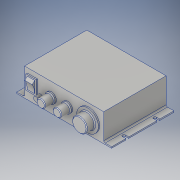
# Autodesk Inventor part: AmpLP2020A
Saved by Autodesk Inventor 2017 (Build 210142000, 142)
## iProperties
Created: 2018-08-06
Part Number: AmpLP2020A
Material: Aluminum 6061
Document SubType Name: Modeling
Designer: Jake
Density: 2.7 g/cm^3
Appearance: Aluminum - Flat
Author: Jake
Autodesk Inventor part; units mm, degrees
ref_plane "YZ Plane" through (0, 0, 0) normal (1, 0, 0) x (0, 1, 0)
sketch "Sketch1" plane through (0, 0, 0) normal (0, 1, 0) x (-1, 0, 0)
  line L0 (70, -46) -> (-70, -46)
  line L1 (-70, -46) -> (-70, 46)
  line L2 (-70, 46) -> (70, 46)
  line L3 (70, 46) -> (70, -46)
  point P0 (0, 0)
  point P1 (0, -46)
  point P2 (-70, 0)
  dimension "d0" = 92
  dimension "d1" = 140
  constraints: 8 end point, 2 midpoint, 2 parallel, 1 horizontal, 1 horizontal alignment, 1 perpendicular, 1 vertical alignment
  measures "d0" distance of L0.end L1.end
  measures "d1" distance of L0.start L0.end
extrude "Extrusion1" add sketch "Sketch1" along normal blind 2
sketch "Sketch2" plane through (0, 2, 0) normal (0, 1, 0) x (1, 0, 0)
  line L0 (70, 46) -> (-70, 46) projected
  line L1 (-70, 46) -> (-70, -46) projected
  line L2 (-70, -46) -> (70, -46) projected
  line L3 (70, -46) -> (70, 46) projected
  line L4 (70, 46) -> (-70, 46) projected
  line L5 (-70, -46) -> (70, -46) projected
  line L6 (-58.5, 46) -> (58.5, 46)
  line L7 (58.5, 46) -> (58.5, -46)
  line L8 (58.5, -46) -> (-58.5, -46)
  line L9 (-58.5, -46) -> (-58.5, 46)
  point P0 (0, 0)
  point P1 (0, 46)
  dimension "d4" = 117
  constraints: 8 end point, 2 midpoint, 2 parallel, 2 point on line, 1 horizontal, 1 perpendicular
  measures "d4" distance between parallel lines of L7 L9
extrude "Extrusion2" add sketch "Sketch2" along normal blind 39 contours L7 L2 L9 L0
fillet "Fillet1" radius 2 2 edges at (58.5, 2, 0) (-58.5, 2, 0)
sketch "Sketch3" plane through (-70, 0, 46) normal (0, 0, 1) x (1, 0, 0)
  line L0 (140, 0) -> (0, 0) projected
  line L1 (140, 0) -> (140, 2) projected
  line L2 (130.5, 2) -> (140, 2) projected
  arc A0 (128.5, 4) -> (130.5, 2) centre (130.5, 4) ccw projected
  line L3 (128.5, 4) -> (128.5, 41) projected
  line L4 (11.5, 41) -> (128.5, 41) projected
  line L5 (11.5, 4) -> (11.5, 41) projected
  arc A1 (9.5, 2) -> (11.5, 4) centre (9.5, 4) ccw projected
  line L6 (0, 2) -> (9.5, 2) projected
  line L7 (0, 0) -> (0, 2) projected
  circle A2 centre (106.5, 20) radius 16
  circle A3 centre (75, 20.5) radius 7.5
  circle A4 centre (51, 20.5) radius 7.5
  circle A5 centre (35, 13.5) radius 3.5
  line L8 (15.5, 34) -> (30.5, 34)
  line L9 (30.5, 34) -> (30.5, 13)
  line L10 (30.5, 13) -> (15.5, 13)
  line L11 (15.5, 13) -> (15.5, 34)
  point P0 (70, 0)
  dimension "d8" = 32
  dimension "d9" = 15
  dimension "d10" = 15
  dimension "d11" = 7
  dimension "d12" = 15
  dimension "d13" = 21
  dimension "d14" = 4
  dimension "d15" = 7
  dimension "d17" = 10
  dimension "d18" = 20
  dimension "d19" = 13
  dimension "d20" = 32
  dimension "d21" = 13
  dimension "d22" = 56
  dimension "d23" = 4
  dimension "d24" = 6
  constraints: 8 end point, 4 centre point, 2 parallel, 1 horizontal, 1 perpendicular
  measures "d8" diameter of A2
  measures "d9" diameter of A3
  measures "d10" diameter of A4
  measures "d11" diameter of A5
  measures "d12" distance of L8.start L8.end
  measures "d13" distance of L10.end L8.start
  measures "d14" distance between parallel lines of L5 L11
  measures "d15" distance between parallel lines of L4 L8
  measures "d17" distance edge to line of A5 L0
  measures "d18" distance edge to line of A5 L5
  measures "d19" distance edge to line of A4 L0
  measures "d20" distance edge to line of A4 L5
  measures "d21" distance edge to line of A3 L0
  measures "d22" distance edge to line of A3 L5
  measures "d23" distance edge to line of A2 L0
  measures "d24" distance edge to line of A2 L3
extrude "Extrusion3" add sketch "Sketch3" along normal blind 2 contours A2 | A3 | A4 | A5 | L8 L9 L10 L11
sketch "Sketch4" plane through (-70, 0, 46) normal (0, 0, 1) x (1, 0, 0)
  circle A0 centre (35, 13.5) radius 3.5 projected
  circle A1 centre (51, 20.5) radius 7.5 projected
  circle A2 centre (75, 20.5) radius 7.5 projected
  circle A3 centre (106.5, 20) radius 16 projected
  circle A4 centre (51, 20.5) radius 6.25
  circle A5 centre (75, 20.5) radius 6.25
  point P0 (70, 0)
  dimension "d28" = 12.5
  dimension "d30" = 12.5
  constraints: 2 centre point, 2 coincident
  measures "d28" diameter of A4
  measures "d30" diameter of A5
extrude "Extrusion4" add sketch "Sketch4" along normal blind 15.7 contours A4 | A5
sketch "Sketch5" plane through (-70, 0, 46) normal (0, 0, 1) x (1, 0, 0)
  circle A0 centre (106.5, 20) radius 16 projected
  circle A1 centre (106.5, 20) radius 10.85
  point P0 (70, 0)
  dimension "d33" = 21.7
  constraints: 1 centre point, 1 coincident
  measures "d33" diameter of A1
extrude "Extrusion5" add sketch "Sketch5" along normal blind 14 contours A1
sketch "Sketch6" plane through (-70, 0, 46) normal (0, 0, 1) x (1, 0, 0)
  circle A0 centre (35, 13.5) radius 3.5 projected
  circle A1 centre (35, 13.5) radius 3.5
  point P0 (70, 0)
  constraints: 1 centre point, 1 coincident, 1 concentric
extrude "Extrusion6" add sketch "Sketch6" along normal blind 6.6
chamfer "Chamfer1" distance 1.25 angle 45 3 edges at (25.65, 20, 48) (-1.25, 20.5, 48) (-25.25, 20.5, 48)
chamfer "Chamfer2" distance 1 angle 45 3 edges at (-25.25, 20.5, 61.7) (-1.25, 20.5, 61.7) (25.65, 20, 60)
ref_plane "Work Plane1" through (-52.5, 13, 46) normal (-1, 0, 0) x (0, 0, 1)
ref_plane "Work Plane2" through (-41.5, 13, 46) normal (1, 0, 0) x (0, 0, -1)
sketch "Sketch7" plane through (-52.5, 13, 46) normal (-1, 0, 0) x (0, 0, 1)
  line L0 (0, 0) -> (0, 21) projected
  line L1 (0, 0) -> (2, 0) projected
  line L2 (2, 21) -> (2, 0) projected
  line L3 (0, 21) -> (2, 21) projected
  line L4 (2, -9) -> (2, 23) projected
  line L5 (2, 19) -> (2, 2)
  line L6 (2, 19) -> (5.6, 15.4)
  arc A0 (5.6, 15.4) -> (2, 2) centre (28.7389, 2) ccw
  point P0 (-46, -13)
  dimension "d46" = 2
  dimension "d47" = 2
  dimension "d48" = 45
  dimension "d49" = 3.6
  constraints: 4 end point, 2 point on circle, 2 point on line, 2 tangent, 1 centre point
  measures "d46" distance from line of L3 L5.start
  measures "d47" distance from line of L1 L5.end
  measures "d48" angle of L2 L6
  measures "d49" distance from line of L2 L6.end
extrude "Extrusion7" add sketch "Sketch7" against normal up to surface (11 mm away) contours L2 L6 A0
sketch "Sketch8" plane through (0, 2, 0) normal (0, 1, 0) x (1, 0, 0)
  line L0 (-60.5, 46) -> (-60.5, -46) projected
  line L1 (-60.5, 46) -> (-70, 46) projected
  line L2 (-70, 46) -> (-70, -46) projected
  line L3 (-70, -46) -> (-60.5, -46) projected
  line L4 (60.5, -46) -> (60.5, 46) projected
  line L5 (60.5, -46) -> (70, -46) projected
  line L6 (70, -46) -> (70, 46) projected
  line L7 (70, 46) -> (60.5, 46) projected
  line L8 (-70, 46) -> (-70, -46) projected
  line L9 (-70, 22.85) -> (-65.15, 22.85) construction
  line L10 (-70, 20.7) -> (-65.15, 20.7)
  line L11 (-65.15, 25) -> (-70, 25)
  arc A0 (-70, 25) -> (-70, 20.7) centre (-70, 22.85) ccw
  arc A1 (-65.15, 20.7) -> (-65.15, 25) centre (-65.15, 22.85) ccw
  line L12 (-70, -22.85) -> (-65.15, -22.85) construction
  line L13 (-70, -25) -> (-65.15, -25)
  line L14 (-65.15, -20.7) -> (-70, -20.7)
  arc A2 (-70, -20.7) -> (-70, -25) centre (-70, -22.85) ccw
  arc A3 (-65.15, -25) -> (-65.15, -20.7) centre (-65.15, -22.85) ccw
  line L15 (70, -22.85) -> (65.15, -22.85) construction
  line L16 (70, -25) -> (65.15, -25)
  line L17 (65.15, -20.7) -> (70, -20.7)
  arc A4 (70, -25) -> (70, -20.7) centre (70, -22.85) ccw
  arc A5 (65.15, -20.7) -> (65.15, -25) centre (65.15, -22.85) ccw
  line L18 (70, 46) -> (70, -46) projected
  line L19 (70, 22.85) -> (65.15, 22.85) construction
  line L20 (70, 20.7) -> (65.15, 20.7)
  line L21 (65.15, 25) -> (70, 25)
  arc A6 (70, 20.7) -> (70, 25) centre (70, 22.85) ccw
  arc A7 (65.15, 25) -> (65.15, 20.7) centre (65.15, 22.85) ccw
  line L22 (70, -46) -> (70, 46) projected
  point P0 (0, 0)
  point P1 (-67.575, 22.85)
  point P2 (-67.575, -22.85)
  point P3 (67.575, -22.85)
  point P4 (67.575, 22.85)
  dimension "d52" = 4.3
  dimension "d54" = 4.3
  dimension "d55" = 4.3
  dimension "d56" = 7
  dimension "d58" = 7
  dimension "d59" = 7
  dimension "d66" = 4.3
  dimension "d67" = 7
  dimension "d68" = 23.15
  dimension "d69" = 23.15
  dimension "d70" = 23.15
  dimension "d71" = 23.15
  constraints: 32 end point, 16 point on circle, 16 tangent, 8 centre point, 4 midpoint, 4 parallel, 4 perpendicular, 4 point on line
  measures "d52" distance between parallel lines of L10 L11
  measures "d54" distance between parallel lines of L13 L14
  measures "d55" distance between parallel lines of L16 L17
  measures "d66" distance between parallel lines of L20 L21
  measures "d68" distance between parallel lines of L9 L1
  measures "d69" distance between parallel lines of L12 L3
  measures "d70" distance between parallel lines of L19 L7
  measures "d71" distance between parallel lines of L15 L5
extrude "Extrusion8" cut sketch "Sketch8" against normal through all contours L11 A1 L10 L2 | L2 A0 | A2 L2 | L2 L14 A3 L13 | L16 A5 L17 L6 | L6 A4 | A6 L6 | L6 L20 A7 L21
equation "\"d10\" = d9"
equation "\"d21\" = d19"
equation "\"d28\" = d27"
equation "\"d30\" = d28"
equation "\"d54\" = d52"
equation "\"d55\" = d52"
equation "\"d58\" = d56"
equation "\"d59\" = d56"
equation "\"d66\" = d52"
equation "\"d67\" = d56"
equation "\"d69\" = d68"
equation "\"d70\" = d68"
equation "\"d71\" = d68"
equation "\"d27\" = 12.5"
body "Solid1"
